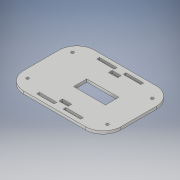
# Autodesk Inventor part: top_plate
Saved by Autodesk Inventor 2017 (Build 210142000, 142)
## iProperties
Created: 2017-06-15
Part Number: top_plate
Material: Generic
Document SubType Name: Modeling
Designer: millerid
Density: 1 g/cm^3
Appearance: Default
Author: millerid
Autodesk Inventor part; units mm, degrees
ref_plane "YZ Plane" through (0, 0, 0) normal (1, 0, 0) x (0, 1, 0)
ref_plane "XZ Plane" through (0, 0, 0) normal (0, 1, 0) x (-1, 0, 0)
ref_plane "XY Plane" through (0, 0, 0) normal (0, 0, 1) x (1, 0, 0)
sketch "Sketch3" plane through (0, 0, 0) normal (0, 1, 0) x (-1, 0, 0)
  line L0 (20, 0) -> (89.97, 0)
  line L1 (109.97, -20) -> (109.97, -60)
  line L2 (89.97, -80) -> (20, -80)
  line L3 (0, -60) -> (0, -20)
  arc A0 (109.97, -20) -> (89.97, 0) centre (89.97, -20) ccw
  arc A1 (89.97, -80) -> (109.97, -60) centre (89.97, -60) ccw
  arc A2 (0, -60) -> (20, -80) centre (20, -60) ccw
  arc A3 (20, 0) -> (0, -20) centre (20, -20) ccw
  line L4 (79.7968, -4.5) -> (60, -4.5)
  line L5 (60, -4.5) -> (60, -7.4718)
  line L6 (60, -7.4718) -> (79.7968, -7.4718)
  line L7 (79.7968, -7.4718) -> (79.7968, -4.5)
  line L8 (30, -4.5) -> (49.7968, -4.5)
  line L9 (49.7968, -4.5) -> (49.7968, -7.4718)
  line L10 (49.7968, -7.4718) -> (30, -7.4718)
  line L11 (30, -7.4718) -> (30, -4.5)
  line L12 (79.7968, -72.5282) -> (60, -72.5282)
  line L13 (60, -72.5282) -> (60, -75.5)
  line L14 (60, -75.5) -> (79.7968, -75.5)
  line L15 (79.7968, -75.5) -> (79.7968, -72.5282)
  line L16 (49.7968, -72.5282) -> (30, -72.5282)
  line L17 (30, -72.5282) -> (30, -75.5)
  line L18 (30, -75.5) -> (49.7968, -75.5)
  line L19 (49.7968, -75.5) -> (49.7968, -72.5282)
  line L20 (60, -10) -> (49.7968, -10)
  line L21 (49.7968, -10) -> (49.7968, -14)
  line L22 (49.7968, -14) -> (60, -14)
  line L23 (60, -14) -> (60, -10)
  line L24 (49.7968, -70) -> (60, -70)
  line L25 (60, -70) -> (60, -66)
  line L26 (60, -66) -> (49.7968, -66)
  line L27 (49.7968, -66) -> (49.7968, -70)
  circle A4 centre (9.9, -65.4) radius 1.5
  circle A5 centre (100.07, -65.4) radius 1.5
  circle A6 centre (9.9, -14.6) radius 1.5
  circle A7 centre (100.07, -14.6) radius 1.5
  line L28 (65.97, -32.5) -> (29.97, -32.5)
  line L29 (29.97, -32.5) -> (29.97, -47.5)
  line L30 (29.97, -47.5) -> (65.97, -47.5)
  line L31 (65.97, -47.5) -> (65.97, -32.5)
  point P0 (0, 0)
  point P1 (109.97, -80)
  point P2 (109.97, 0)
  point P3 (0, -80)
  dimension "d0" = 109.97
  dimension "d1" = 80
  dimension "d2" = 20
  dimension "d3" = 19.7968
  dimension "d4" = 2.9718
  dimension "d5" = 4.5
  dimension "d7" = 19.7968
  dimension "d8" = 30
  dimension "d9" = 2.9718
  dimension "d10" = 4.5
  dimension "d11" = 4
  dimension "d12" = 10
  dimension "d13" = 4
  dimension "d14" = 10
  dimension "d15" = 3
  dimension "d16" = 3
  dimension "d17" = 3
  dimension "d22" = 9.9
  dimension "d23" = 9.9
  dimension "d24" = 9.9
  dimension "d25" = 9.9
  dimension "d26" = 14.6
  dimension "d27" = 14.6
  dimension "d28" = 14.6
  dimension "d29" = 14.6
  dimension "d30" = 36
  dimension "d31" = 15
  dimension "d32" = 44
  dimension "d33" = 32.5
  dimension "d36" = 10.2032
  constraints: 64 end point, 16 parallel, 11 collinear, 9 point on line, 8 centre point, 8 horizontal, 8 perpendicular, 8 point on circle, 8 tangent, 3 equal radius
  measures "d0" distance of point (109.97, -80) point (0, -80)
  measures "d1" distance of point (109.97, 0) point (109.97, -80)
  measures "d2" radius of A0
  measures "d3" distance of L6.end L5.end
  measures "d4" distance of L5.end L4.end
  measures "d5" distance between parallel lines of L0 L4
  measures "d7" distance of L9.end L10.end
  measures "d8" distance between parallel lines of L3 L11
  measures "d9" distance of L13.end L12.end
  measures "d10" distance between parallel lines of L2 L14
  measures "d11" distance of L21.end L20.end
  measures "d12" distance between parallel lines of L0 L20
  measures "d13" distance of L25.end L24.end
  measures "d14" distance between parallel lines of L2 L24
  measures "d15" diameter of A4
  measures "d16" diameter of A5
  measures "d17" diameter of A6
  measures "d22" distance from line of L1 A7.centre
  measures "d23" distance from line of L1 A5.centre
  measures "d24" distance from line of L3 A6.centre
  measures "d25" distance from line of L3 A4.centre
  measures "d26" distance from line of L0 A7.centre
  measures "d27" distance from line of L2 A5.centre
  measures "d28" distance from line of L0 A6.centre
  measures "d29" distance from line of L2 A4.centre
  measures "d30" distance of L30.end L29.end
  measures "d31" distance of L29.end L28.end
  measures "d32" distance between parallel lines of L1 L31
  measures "d33" distance between parallel lines of L0 L28
  measures "d36" distance between parallel lines of L9 L5
extrude "Extrusion1" add sketch "Sketch3" along normal blind 3.175
equation "\"d3\" = d7"
equation "\"d9\" = d4"
equation "\"d10\" = d5"
equation "\"d14\" = d12"
equation "\"d23\" = d22"
equation "\"d24\" = d22"
equation "\"d25\" = d22"
equation "\"d27\" = d26"
equation "\"d28\" = d26"
equation "\"d29\" = d26"
equation "\"d33\" = -0.5 * d31 + 0.5 * d1"
body "Solid1"
